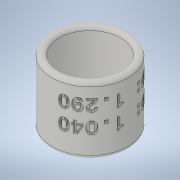
# Autodesk Inventor part: LargeFinderEyePieceCover
Saved by Autodesk Inventor 2021.1 (Build 251245000, 245)
## iProperties
Created: 2018-09-01
Part Number: LargeFinderEyePieceCover
Material: Generic
Document SubType Name: Modeling
Designer: steele
Density: 1 g/cm^3
Appearance: Default
Author: steele
Autodesk Inventor part; units mm, degrees
ref_plane "XZ Plane" through (0, 0, 0) normal (0, 1, 0) x (-1, 0, 0)
ref_plane "XY Plane" through (0, 0, 0) normal (0, 0, 1) x (1, 0, 0)
sketch "Sketch1" plane through (0, 0, 0) normal (0, 1, 0) x (-1, 0, 0)
  circle A0 centre (0, 0) radius 16.383
  dimension "d0" = 32.766
  constraints: 1 centre point, 1 coincident
  measures "d0" diameter of A0
extrude "Extrusion1" add sketch "Sketch1" along normal blind 3.175
sketch "Sketch2" plane through (0, 3.175, 0) normal (0, 1, 0) x (1, 0, 0)
  circle A0 centre (0, 0) radius 16.383
  circle A1 centre (0, 0) radius 13.208
  dimension "d3" = 32.766
  dimension "d4" = 26.416
  constraints: 2 centre point, 2 coincident
  measures "d3" diameter of A0
  measures "d4" diameter of A1
extrude "Extrusion2" add sketch "Sketch2" along normal blind 25.4
ref_plane "Work Plane1" through (16.383, 0, 0) normal (1, 0, 0) x (0, 1, 0)
sketch "Sketch3" plane through (16.383, 0, 0) normal (1, 0, 0) x (0, 1, 0)
  line L0 (0, 16.383) -> (28.575, 16.383) construction
  line L1 (14.2875, 16.383) -> (14.2875, -16.3747) construction
  line L2 (3.175, -13.208) -> (28.575, -13.208) construction
  line L3 (10.082, -14.707) -> (10.082, -15.6373)
  line L4 (10.082, -15.6373) -> (9.2075, -15.6373)
  line L5 (9.2075, -15.6373) -> (9.2075, -12.7093)
  line L6 (9.2075, -12.7093) -> (10.082, -12.7093)
  line L7 (10.082, -12.7093) -> (10.082, -13.6396)
  line L8 (10.082, -13.6396) -> (13.4087, -13.6396)
  line L9 (13.4087, -13.6396) -> (13.4087, -12.7093)
  line L10 (13.4087, -12.7093) -> (14.2875, -12.7093)
  line L11 (14.2875, -12.7093) -> (14.2875, -15.6373)
  line L12 (14.2875, -15.6373) -> (13.4087, -15.6373)
  line L13 (13.4087, -15.6373) -> (13.4087, -14.707)
  line L14 (13.4087, -14.707) -> (10.082, -14.707)
  spline S0 degree 2 poles (9.2075, -9.7642) (9.2075, -8.8383) (10.5021, -7.8737) (11.7454, -7.8737) knots 0 0 0 1 2 2 2
  spline S1 degree 2 poles (11.7454, -7.8737) (13.0057, -7.8737) (14.2875, -8.8297) (14.2875, -9.7642) knots 0 0 0 1 2 2 2
  line L15 (14.2875, -9.7642) -> (14.2875, -11.4576)
  line L16 (14.2875, -11.4576) -> (9.2075, -11.4576)
  line L17 (9.2075, -11.4576) -> (9.2075, -9.7642)
  line L18 (10.1506, -9.7642) -> (10.1506, -10.3815)
  line L19 (10.1506, -10.3815) -> (13.3358, -10.3815)
  line L20 (13.3358, -10.3815) -> (13.3358, -9.7642)
  spline S2 degree 2 poles (13.3358, -9.7642) (13.3358, -9.3484) (12.5942, -8.9711) (11.7454, -8.9711) knots 0 0 0 1 2 2 2
  spline S3 degree 2 poles (11.7454, -8.9711) (10.9566, -8.9711) (10.1506, -9.3741) (10.1506, -9.7642) knots 0 0 0 1 2 2 2
  line L21 (12.9414, -6.0217) -> (12.9414, -4.6757)
  line L22 (12.9414, -4.6757) -> (14.2875, -4.6757)
  line L23 (14.2875, -4.6757) -> (14.2875, -6.0217)
  line L24 (14.2875, -6.0217) -> (12.9414, -6.0217)
  line L25 (10.3564, -6.0217) -> (10.3564, -4.6757)
  line L26 (10.3564, -4.6757) -> (11.7025, -4.6757)
  line L27 (11.7025, -4.6757) -> (11.7025, -6.0217)
  line L28 (11.7025, -6.0217) -> (10.3564, -6.0217)
  line L29 (10.7894, 3.268) -> (10.7894, 2.0462)
  line L30 (10.7894, 2.0462) -> (10.0692, 2.0462)
  line L31 (10.0692, 2.0462) -> (10.0692, 2.0977)
  spline S4 degree 2 poles (10.0692, 2.0977) (10.0692, 2.8007) (9.6705, 3.3966) (9.1689, 3.4566) knots 0 0 0 1 2 2 2
  line L32 (9.1689, 3.4566) -> (9.1689, 4.2797)
  line L33 (9.1689, 4.2797) -> (14.2875, 4.2797)
  line L34 (14.2875, 4.2797) -> (14.2875, 3.268)
  line L35 (14.2875, 3.268) -> (10.7894, 3.268)
  line L36 (12.9414, 7.212) -> (12.9414, 8.5581)
  line L37 (12.9414, 8.5581) -> (14.2875, 8.5581)
  line L38 (14.2875, 8.5581) -> (14.2875, 7.212)
  line L39 (14.2875, 7.212) -> (12.9414, 7.212)
  spline S5 degree 2 poles (11.7325, 10.4443) (10.4721, 10.4443) (9.1689, 11.3831) (9.1689, 12.2963) knots 0 0 0 1 2 2 2
  spline S6 degree 2 poles (9.1689, 12.2963) (9.1689, 13.2222) (10.485, 14.1439) (11.8097, 14.1439) knots 0 0 0 1 2 2 2
  spline S7 degree 2 poles (11.8097, 14.1439) (13.13, 14.1439) (14.429, 13.2308) (14.429, 12.2963) knots 0 0 0 1 2 2 2
  spline S8 degree 2 poles (14.429, 12.2963) (14.429, 11.3574) (13.1043, 10.4443) (11.7325, 10.4443) knots 0 0 0 1 2 2 2
  spline S9 degree 2 poles (10.0263, 12.2877) (10.0263, 11.889) (10.8623, 11.5075) (11.7368, 11.5075) knots 0 0 0 1 2 2 2
  spline S10 degree 2 poles (11.7368, 11.5075) (12.7185, 11.5075) (13.5759, 11.8761) (13.5759, 12.2877) knots 0 0 0 1 2 2 2
  spline S11 degree 2 poles (13.5759, 12.2877) (13.5759, 12.6992) (12.7271, 13.0808) (11.8011, 13.0808) knots 0 0 0 1 2 2 2
  spline S12 degree 2 poles (11.8011, 13.0808) (10.8708, 13.0808) (10.0263, 12.6992) (10.0263, 12.2877) knots 0 0 0 1 2 2 2
  line L40 (13.1815, 16.9519) -> (13.1815, 14.8041)
  line L41 (13.1815, 14.8041) -> (12.2812, 14.8041)
  line L42 (12.2812, 14.8041) -> (9.3147, 16.6818)
  line L43 (9.3147, 16.6818) -> (9.3147, 17.9593)
  line L44 (9.3147, 17.9593) -> (12.367, 17.9593)
  line L45 (12.367, 17.9593) -> (12.367, 18.5552)
  line L46 (12.367, 18.5552) -> (13.1815, 18.5552)
  line L47 (13.1815, 18.5552) -> (13.1815, 17.9593)
  line L48 (13.1815, 17.9593) -> (14.2875, 17.9593)
  line L49 (14.2875, 17.9593) -> (14.2875, 16.9519)
  line L50 (14.2875, 16.9519) -> (13.1815, 16.9519)
  line L51 (12.3927, 15.5843) -> (12.3927, 16.9819)
  line L52 (12.3927, 16.9819) -> (10.2021, 16.9819)
  line L53 (10.2021, 16.9819) -> (12.3927, 15.5843)
  spline S13 degree 2 poles (11.7325, 19.2668) (10.4721, 19.2668) (9.1689, 20.2056) (9.1689, 21.1187) knots 0 0 0 1 2 2 2
  spline S14 degree 2 poles (9.1689, 21.1187) (9.1689, 22.0447) (10.485, 22.9664) (11.8097, 22.9664) knots 0 0 0 1 2 2 2
  spline S15 degree 2 poles (11.8097, 22.9664) (13.13, 22.9664) (14.429, 22.0533) (14.429, 21.1187) knots 0 0 0 1 2 2 2
  spline S16 degree 2 poles (14.429, 21.1187) (14.429, 20.1799) (13.1043, 19.2668) (11.7325, 19.2668) knots 0 0 0 1 2 2 2
  spline S17 degree 2 poles (10.0263, 21.1102) (10.0263, 20.7115) (10.8623, 20.33) (11.7368, 20.33) knots 0 0 0 1 2 2 2
  spline S18 degree 2 poles (11.7368, 20.33) (12.7185, 20.33) (13.5759, 20.6986) (13.5759, 21.1102) knots 0 0 0 1 2 2 2
  spline S19 degree 2 poles (13.5759, 21.1102) (13.5759, 21.5217) (12.7271, 21.9033) (11.8011, 21.9033) knots 0 0 0 1 2 2 2
  spline S20 degree 2 poles (11.8011, 21.9033) (10.8708, 21.9033) (10.0263, 21.5217) (10.0263, 21.1102) knots 0 0 0 1 2 2 2
  spline S21 degree 2 poles (20.1171, -16.0531) (18.8997, -16.0531) (17.4893, -15.0371) (17.4893, -14.1712) knots 0 0 0 1 2 2 2
  spline S22 degree 2 poles (17.4893, -14.1712) (17.4893, -13.2924) (18.9168, -12.2892) (20.1686, -12.2892) knots 0 0 0 1 2 2 2
  spline S23 degree 2 poles (20.1686, -12.2892) (21.4247, -12.2892) (22.8522, -13.2924) (22.8522, -14.1712) knots 0 0 0 1 2 2 2
  spline S24 degree 2 poles (22.8522, -14.1712) (22.8522, -15.0586) (21.4161, -16.0531) (20.1171, -16.0531) knots 0 0 0 1 2 2 2
  spline S25 degree 2 poles (18.4324, -14.1755) (18.4324, -14.5484) (19.2726, -14.9643) (20.0443, -14.9643) knots 0 0 0 1 2 2 2
  spline S26 degree 2 poles (20.0443, -14.9643) (21.0003, -14.9643) (21.8919, -14.5742) (21.8919, -14.154) knots 0 0 0 1 2 2 2
  spline S27 degree 2 poles (21.8919, -14.154) (21.8919, -13.7639) (21.0646, -13.3867) (20.1814, -13.3867) knots 0 0 0 1 2 2 2
  spline S28 degree 2 poles (20.1814, -13.3867) (19.2983, -13.3867) (18.4324, -13.7768) (18.4324, -14.1755) knots 0 0 0 1 2 2 2
  spline S29 degree 2 poles (17.6307, -9.7642) (17.6307, -8.8383) (18.9254, -7.8737) (20.1686, -7.8737) knots 0 0 0 1 2 2 2
  spline S30 degree 2 poles (20.1686, -7.8737) (21.4289, -7.8737) (22.7107, -8.8297) (22.7107, -9.7642) knots 0 0 0 1 2 2 2
  line L54 (22.7107, -9.7642) -> (22.7107, -11.4576)
  line L55 (22.7107, -11.4576) -> (17.6307, -11.4576)
  line L56 (17.6307, -11.4576) -> (17.6307, -9.7642)
  line L57 (18.5739, -9.7642) -> (18.5739, -10.3815)
  line L58 (18.5739, -10.3815) -> (21.759, -10.3815)
  line L59 (21.759, -10.3815) -> (21.759, -9.7642)
  spline S31 degree 2 poles (21.759, -9.7642) (21.759, -9.3484) (21.0174, -8.9711) (20.1686, -8.9711) knots 0 0 0 1 2 2 2
  spline S32 degree 2 poles (20.1686, -8.9711) (19.3798, -8.9711) (18.5739, -9.3741) (18.5739, -9.7642) knots 0 0 0 1 2 2 2
  line L60 (18.7796, -6.0217) -> (18.7796, -4.6757)
  line L61 (18.7796, -4.6757) -> (20.1257, -4.6757)
  line L62 (20.1257, -4.6757) -> (20.1257, -6.0217)
  line L63 (20.1257, -6.0217) -> (18.7796, -6.0217)
  line L64 (21.3646, -6.0217) -> (21.3646, -4.6757)
  line L65 (21.3646, -4.6757) -> (22.7107, -4.6757)
  line L66 (22.7107, -4.6757) -> (22.7107, -6.0217)
  line L67 (22.7107, -6.0217) -> (21.3646, -6.0217)
  line L68 (19.2126, 3.268) -> (19.2126, 2.0462)
  line L69 (19.2126, 2.0462) -> (18.4924, 2.0462)
  line L70 (18.4924, 2.0462) -> (18.4924, 2.0977)
  spline S33 degree 2 poles (18.4924, 2.0977) (18.4924, 2.8007) (18.0937, 3.3966) (17.5921, 3.4566) knots 0 0 0 1 2 2 2
  line L71 (17.5921, 3.4566) -> (17.5921, 4.2797)
  line L72 (17.5921, 4.2797) -> (22.7107, 4.2797)
  line L73 (22.7107, 4.2797) -> (22.7107, 3.268)
  line L74 (22.7107, 3.268) -> (19.2126, 3.268)
  line L75 (21.3646, 7.212) -> (21.3646, 8.5581)
  line L76 (21.3646, 8.5581) -> (22.7107, 8.5581)
  line L77 (22.7107, 8.5581) -> (22.7107, 7.212)
  line L78 (22.7107, 7.212) -> (21.3646, 7.212)
  line L79 (19.4227, 11.4603) -> (19.4227, 10.5172)
  line L80 (19.4227, 10.5172) -> (19.4012, 10.5172)
  spline S34 degree 2 poles (19.4012, 10.5172) (18.5567, 10.5172) (17.5921, 11.456) (17.5921, 12.2791) knots 0 0 0 1 2 2 2
  spline S35 degree 2 poles (17.5921, 12.2791) (17.5921, 13.1108) (18.4452, 14.0753) (19.1654, 14.0753) knots 0 0 0 1 2 2 2
  spline S36 degree 2 poles (19.1654, 14.0753) (19.6799, 14.0753) (20.4472, 13.5695) (20.9059, 12.8664) knots 0 0 0 1 2 2 2
  spline S37 degree 2 poles (20.9059, 12.8664) (21.0045, 12.725) (21.1632, 12.472) knots 0 0 0 1 1 1
  spline S38 degree 2 poles (21.1632, 12.472) (21.6047, 11.7775) (21.8362, 11.6961) knots 0 0 0 1 1 1
  line L81 (21.8362, 11.6961) -> (21.8362, 14.0239)
  line L82 (21.8362, 14.0239) -> (22.7107, 14.0239)
  line L83 (22.7107, 14.0239) -> (22.7107, 10.4315)
  spline S39 degree 2 poles (22.7107, 10.4315) (22.012, 10.4443) (21.0731, 11.0102) (20.5801, 11.7433) knots 0 0 0 1 2 2 2
  spline S40 degree 2 poles (20.5801, 11.7433) (20.503, 11.8547) (20.3658, 12.0691) knots 0 0 0 1 1 1
  spline S41 degree 2 poles (20.3658, 12.0691) (19.757, 13.0293) (19.1826, 13.0293) knots 0 0 0 1 1 1
  spline S42 degree 2 poles (19.1826, 13.0293) (18.8482, 13.0293) (18.4495, 12.6178) (18.4495, 12.2663) knots 0 0 0 1 2 2 2
  spline S43 degree 2 poles (18.4495, 12.2663) (18.4495, 11.8847) (18.934, 11.4603) (19.3798, 11.4603) knots 0 0 0 1 2 2 2
  line L84 (19.3798, 11.4603) -> (19.4227, 11.4603)
  line L85 (21.5576, 14.967) -> (21.5533, 16.0087)
  spline S44 degree 2 poles (21.5533, 16.0087) (21.7933, 16.0387) (22.0548, 16.3517) (22.0548, 16.6089) knots 0 0 0 1 2 2 2
  spline S45 degree 2 poles (22.0548, 16.6089) (22.0548, 17.0119) (21.3989, 17.4277) (20.7045, 17.4577) knots 0 0 0 1 2 2 2
  spline S46 degree 2 poles (20.7045, 17.4577) (20.8802, 17.2862) (21.0646, 16.789) (21.0646, 16.4889) knots 0 0 0 1 2 2 2
  spline S47 degree 2 poles (21.0646, 16.4889) (21.0646, 15.7344) (20.1557, 14.8255) (19.3927, 14.8255) knots 0 0 0 1 2 2 2
  spline S48 degree 2 poles (19.3927, 14.8255) (18.5867, 14.8255) (17.5921, 15.8115) (17.5921, 16.6218) knots 0 0 0 1 2 2 2
  spline S49 degree 2 poles (17.5921, 16.6218) (17.5921, 17.552) (18.8868, 18.5294) (20.1214, 18.5294) knots 0 0 0 1 2 2 2
  spline S50 degree 2 poles (20.1214, 18.5294) (21.4504, 18.5294) (22.8651, 17.4877) (22.8651, 16.5103) knots 0 0 0 1 2 2 2
  spline S51 degree 2 poles (22.8651, 16.5103) (22.8651, 15.8373) (22.1491, 15.0013) (21.5576, 14.967) knots 0 0 0 1 2 2 2
  spline S52 degree 2 poles (20.2372, 16.6646) (20.2372, 17.029) (19.7785, 17.4449) (19.3712, 17.4449) knots 0 0 0 1 2 2 2
  spline S53 degree 2 poles (19.3712, 17.4449) (18.9297, 17.4449) (18.4195, 17.0076) (18.4195, 16.6261) knots 0 0 0 1 2 2 2
  spline S54 degree 2 poles (18.4195, 16.6261) (18.4195, 16.2788) (18.9168, 15.8673) (19.3412, 15.8673) knots 0 0 0 1 2 2 2
  spline S55 degree 2 poles (19.3412, 15.8673) (19.7656, 15.8673) (20.2372, 16.2831) (20.2372, 16.6646) knots 0 0 0 1 2 2 2
  spline S56 degree 2 poles (20.1557, 19.2668) (18.8954, 19.2668) (17.5921, 20.2056) (17.5921, 21.1187) knots 0 0 0 1 2 2 2
  spline S57 degree 2 poles (17.5921, 21.1187) (17.5921, 22.0447) (18.9082, 22.9664) (20.2329, 22.9664) knots 0 0 0 1 2 2 2
  spline S58 degree 2 poles (20.2329, 22.9664) (21.5533, 22.9664) (22.8522, 22.0533) (22.8522, 21.1187) knots 0 0 0 1 2 2 2
  spline S59 degree 2 poles (22.8522, 21.1187) (22.8522, 20.1799) (21.5275, 19.2668) (20.1557, 19.2668) knots 0 0 0 1 2 2 2
  spline S60 degree 2 poles (18.4495, 21.1102) (18.4495, 20.7115) (19.2855, 20.33) (20.16, 20.33) knots 0 0 0 1 2 2 2
  spline S61 degree 2 poles (20.16, 20.33) (21.1417, 20.33) (21.9991, 20.6986) (21.9991, 21.1102) knots 0 0 0 1 2 2 2
  spline S62 degree 2 poles (21.9991, 21.1102) (21.9991, 21.5217) (21.1503, 21.9033) (20.2243, 21.9033) knots 0 0 0 1 2 2 2
  spline S63 degree 2 poles (20.2243, 21.9033) (19.2941, 21.9033) (18.4495, 21.5217) (18.4495, 21.1102) knots 0 0 0 1 2 2 2
  point P0 (0, 0)
  constraints: 2 end point, 1 midpoint, 1 perpendicular, 1 vertical
emboss "Emboss1" sketch "Sketch3" operation cut depth 1.27 direction (1, 0, 0) wrap yes faces at (-16.1708, 10.5833, -2.628)
fillet "Fillet1" radius 1.5875 1 edges at (16.383, 0, 0)
fillet "Fillet2" radius 1.5875 2 edges at (-13.208, 28.575, 0) (-16.383, 28.575, 0)
equation "\"d0\" = coverOD"
equation "\"d1\" = wallThickness"
equation "\"d3\" = coverOD"
equation "\"d4\" = eypPieceCoverID"
equation "\"d7\" = textDepth"
equation "\"d9\" = filletRadius"
equation "\"d10\" = filletRadius"
equation "\"wallThickness\" = 3.175"
equation "\"coverOD\" = eypPieceCoverID + 2 * wallThickness"
equation "\"eypPieceCoverID\" = 26.416"
equation "\"textDepth\" = 1.27"
equation "\"filletRadius\" = 1.5875"
body "Solid1"
